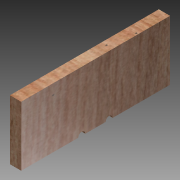
# Autodesk Inventor part: Robot-Base-Support
Saved by Autodesk Inventor 2012 (Build 160160000, 160)
## iProperties
Created: 2013-07-14
Part Number: Robot-Base-Support
Material: Wood (Birch)
Document SubType Name: Modeling
Designer: joe_000
Density: 0.55 g/cm^3
Mass: 79.1257 g
Surface Area: 287.635 cm^2
Volume: 143.865 cm^3
Author: joe_000
Autodesk Inventor part; units mm, degrees
ref_plane "YZ Plane" through (0, 0, 0) normal (1, 0, 0) x (0, 1, 0)
ref_plane "XZ Plane" through (0, 0, 0) normal (0, 1, 0) x (-1, 0, 0)
ref_plane "XY Plane" through (0, 0, 0) normal (0, 0, 1) x (1, 0, 0)
sketch "Sketch1" plane through (0, 0, 0) normal (0, 0, 1) x (1, 0, 0)
  line L0 (0, 0) -> (12.7, 0)
  line L1 (12.7, 0) -> (12.7, 67.5875)
  line L2 (12.7, 67.5875) -> (0, 67.5875)
  line L3 (0, 67.5875) -> (0, 0)
  dimension "d0" = 67.5875
  dimension "d1" = 12.7
  constraints: 8 end point, 2 parallel, 1 horizontal, 1 perpendicular
  measures "d0" distance of L0.end L1.end
  measures "d1" distance of L1.end L2.end
extrude "Extrusion1" add sketch "Sketch1" along normal blind 168.3364
sketch "Sketch2" plane through (12.7, 0, 0) normal (1, 0, 0) x (0, 0, -1)
  line L0 (0, 0) -> (-168.3364, 0) projected
  line L1 (-99.8382, 5.715) -> (-99.8382, 5.715)
  line L2 (-168.3364, 67.5875) -> (-168.3364, 0) projected
  circle A0 centre (-99.8382, 0) radius 3.9688
  circle A1 centre (-68.8382, 0) radius 3.9688
  point P0 (-103.0132, 0)
  dimension "d9" = 7.9375
  dimension "d10" = 31
  dimension "d11" = 68.4982
  constraints: 3 point on line, 2 centre point, 2 end point, 1 equal radius
  measures "d9" diameter of A0
  measures "d10" distance of A1.centre A0.centre
  measures "d11" distance from line of A0.centre L2
extrude "Extrusion3" cut sketch "Sketch2" against normal through all
equation "\"d0\" = BaseSupportHeight"
equation "\"d1\" = BaseSupportThickness"
equation "\"d2\" = BaseSideLength"
equation "\"d10\" = HoleSpacing"
equation "\"BaseSupportHeight\" = 67.5875"
equation "\"BaseSupportThickness\" = 12.7"
equation "\"BaseSideLength\" = 168.336392"
equation "\"HoleSpacing\" = 31"
body "Solid1"
